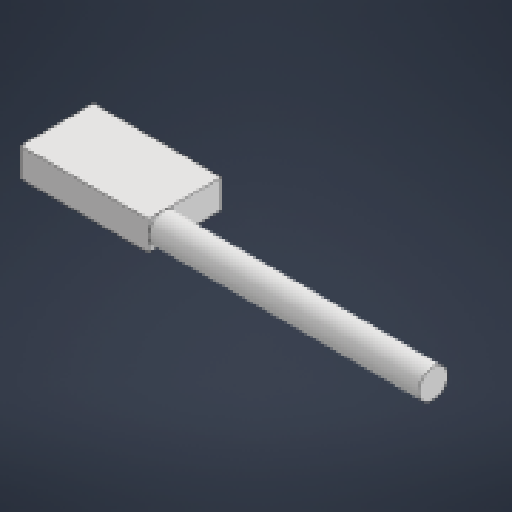
# Autodesk Inventor part: telementry
Saved by Autodesk Inventor 2026.2 (Build 302298000, 298)
## iProperties
Created: 2026-01-10
Part Number: telementry
Material: 一般
Document SubType Name: Modeling
Designer: gavin
Density: 1 g/cm^3
Appearance: 預設
Author: gavin
Autodesk Inventor part; units mm, degrees
ref_plane "YZ Plane" through (0, 0, 0) normal (1, 0, 0) x (0, 1, 0)
ref_plane "XZ Plane" through (0, 0, 0) normal (0, 1, 0) x (-1, 0, 0)
ref_plane "XY Plane" through (0, 0, 0) normal (0, 0, 1) x (1, 0, 0)
sketch "草圖1" plane through (0, 0, 0) normal (0, 1, 0) x (-1, 0, 0)
  line L0 (-23.7, 13.54) -> (23.7, 13.54)
  line L1 (23.7, 13.54) -> (23.7, -13.54)
  line L2 (23.7, -13.54) -> (-23.7, -13.54)
  line L3 (-23.7, -13.54) -> (-23.7, 13.54)
  line L4 (-23.7, 13.54) -> (23.7, -13.54) construction
  line L5 (23.7, 13.54) -> (-23.7, -13.54) construction
  point P0 (0, 0)
  dimension "d0" = 47.4
  dimension "d1" = 27.08
  constraints: 12 end point, 2 midpoint, 2 parallel, 1 horizontal, 1 perpendicular
  measures "d0" distance of L1.end L2.end
  measures "d1" distance of L0.end L1.end
extrude "擠出1" add sketch "草圖1" along normal blind 10.7
sketch "草圖2" plane through (23.7, 0, 13.54) normal (1, 0, 0) x (0, 0, -1)
  circle A0 centre (5.35, 5.35) radius 5.35
  line L0 (27.08, 10.7) -> (0, 10.7) projected
  line L1 (0, 0) -> (0, 10.7) projected
  point P0 (13.54, 0)
  constraints: 2 tangent, 1 centre point
extrude "擠出2" add sketch "草圖2" along normal blind 100 contours A0
